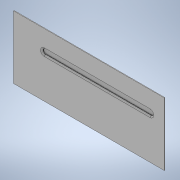
# Autodesk Inventor part: Ambutisare
Saved by Autodesk Inventor 2022 (Build 260153000, 153)
## iProperties
Created: 2022-04-12
Part Number: Ambutisare
Material: Generic
Document SubType Name: Sheet Metal
Designer: Janina
Density: 1 g/cm^3
Sheet Metal Rule: Default_mm
Appearance: Default
Author: Janina
Autodesk Inventor part; units mm, degrees
ref_plane "YZ Plane" through (0, 0, 0) normal (1, 0, 0) x (0, 1, 0)
ref_plane "XZ Plane" through (0, 0, 0) normal (0, 1, 0) x (-1, 0, 0)
ref_plane "XY Plane" through (0, 0, 0) normal (0, 0, 1) x (1, 0, 0)
sketch "Sketch1" plane through (0, 0, 0) normal (0, 0, 1) x (1, 0, 0)
  line L0 (-84.7059, 23.5294) -> (35.2941, 23.5294)
  line L1 (35.2941, 23.5294) -> (35.2941, -26.4706)
  line L2 (35.2941, -26.4706) -> (-84.7059, -26.4706)
  line L3 (-84.7059, -26.4706) -> (-84.7059, 23.5294)
  point P0 (0, 0)
  dimension "d0" = 50
  dimension "d1" = 120
  measures "d0" distance of L0.end L1.end
  measures "d1" distance of L0.start L0.end
extrude "Plate1" add sketch "Sketch1" along normal blind 0.5
sketch "Sketch4" plane through (0, 0, 0.5) normal (0, 0, 1) x (1, 0, 0)
  line L0 (-63.1034, 10.3448) -> (26.8966, 10.3448)
  line L1 (26.8966, 10.3448) -> (26.8966, 4.3448)
  line L2 (26.8966, 4.3448) -> (-63.1034, 4.3448)
  line L3 (-63.1034, 4.3448) -> (-63.1034, 10.3448)
  line L4 (35.2941, 23.5294) -> (35.2941, -26.4706) projected
  line L5 (-84.7059, 23.5294) -> (35.2941, 23.5294) projected
  line L6 (-84.7059, -26.4706) -> (-84.7059, 23.5294) projected
  line L7 (35.2941, -26.4706) -> (-84.7059, -26.4706) projected
  line L8 (25.8966, 9.3448) -> (-62.1034, 9.3448)
  line L9 (-62.1034, 9.3448) -> (-62.1034, 5.3448)
  line L10 (-62.1034, 5.3448) -> (25.8966, 5.3448)
  line L11 (25.8966, 5.3448) -> (25.8966, 9.3448)
  point P0 (0, 0)
  point P1 (-18.1034, 7.3448)
  dimension "d11" = 90
  dimension "d12" = 6
  dimension "d13" = 45
  dimension "d16" = 1
  constraints: 16 end point, 4 parallel, 2 perpendicular, 1 horizontal, 3 other
  measures "d11" distance of L0.start L0.end
  measures "d12" distance of L2.end L0.start
  measures "d13" distance from line of L3 point (-18.103, 7.345)
  measures "d16" distance between parallel lines of L0 L8
extrude "Extrusion3" add sketch "Sketch4" against normal blind 1.8 contours L0 L1 L2 L3 | L11 L10 L9 L8
extrude "Extrusion4" cut sketch "Sketch4" against normal blind 1.4 contours L11 L10 L9 L8
fillet "Fillet1" radius 2 4 edges at (25.8966, 9.3448, -0.2) (25.8966, 5.3448, -0.2) (-62.1034, 5.3448, -0.2) (-62.1034, 9.3448, -0.2)
fillet "Fillet2" radius 3 4 edges at (26.8966, 4.3448, -0.65) (26.8966, 10.3448, -0.65) (-63.1034, 10.3448, -0.65) (-63.1034, 4.3448, -0.65)
fillet "Fillet3" radius 1 16 edges at (25.3108, 8.7591, 0.5) (25.8966, 7.3448, 0.5) (25.3108, 5.9306, 0.5) (-18.1034, 5.3448, 0.5) (-61.5177, 8.7591, 0.5) (-62.1034, 7.3448, 0.5) (-61.5177, 5.9306, 0.5) (-18.1034, 9.3448, 0.5) (26.0179, 9.4662, -1.3) (26.0179, 5.2235, -1.3) (26.8966, 7.3448, -1.3) (-18.1034, 4.3448, -1.3) (-63.1034, 7.3448, -1.3) (-62.2248, 9.4662, -1.3) (-62.2248, 5.2235, -1.3) (-18.1034, 10.3448, -1.3)
fillet "Fillet4" radius 0.2 8 edges at (25.3108, 8.7591, -0.9) (25.8966, 7.3448, -0.9) (25.3108, 5.9306, -0.9) (-18.1034, 5.3448, -0.9) (-61.5177, 8.7591, -0.9) (-62.1034, 7.3448, -0.9) (-61.5177, 5.9306, -0.9) (-18.1034, 9.3448, -0.9)
equation "\"d11\" = LT_A"
equation "\"d12\" = LG_A"
equation "\"d13\" = 0.5 * d11"
equation "\"d16\" = Thickness_Copy"
equation "\"d2\" = Thickness"
equation "\"BendRadius\" = Thickness"
equation "\"BendReliefWidth\" = Thickness"
equation "\"BendReliefDepth\" = 0.5 * Thickness"
equation "\"CornerReliefSize\" = 4 * Thickness"
equation "\"MinimumRemnant\" = 2 * Thickness"
equation "\"TransitionRadius\" = BendRadius"
equation "\"JacobiRadiusSize\" = BendRadius"
equation "\"GapSize\" = Thickness"
equation "\"Thickness_Copy\" = 1"
equation "\"LT_A\" = 90"
equation "\"LG_A\" = 6"
equation "\"Thickness\" = 0.5"
body "Solid1"
